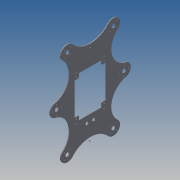
# Autodesk Inventor part: BaseAtas
Saved by Autodesk Inventor 2014 (Build 180170000, 170)
## iProperties
Created: 2014-12-20
Part Number: BaseAtas
Material: Generic
Document SubType Name: Modeling
Designer: I Was ME
Density: 1 g/cm^3
Appearance: Default
Author: I Was ME
Autodesk Inventor part; units mm, degrees
ref_plane "YZ Plane" through (0, 0, 0) normal (1, 0, 0) x (0, 1, 0)
ref_plane "XZ Plane" through (0, 0, 0) normal (0, 1, 0) x (-1, 0, 0)
ref_plane "XY Plane" through (0, 0, 0) normal (0, 0, 1) x (1, 0, 0)
sketch "Sketch1" plane through (0, 0, 0) normal (1, 0, 0) x (0, 1, 0)
  line L0 (0.007, 157.8334) -> (0.007, 7.1531) construction
  line L1 (42.757, 164.9919) -> (42.757, -0.0081) construction
  line L2 (0.007, -0.0081) -> (0.007, 164.9919) construction
  line L3 (-42.743, -0.0081) -> (-42.743, 164.9919) construction
  line L4 (-42.743, 164.9919) -> (42.757, 164.9919) construction
  line L5 (-51.5818, 156.1531) -> (-62.7081, 95.15) construction
  arc A0 (-62.7081, 95.15) -> (-51.5818, 156.1531) centre (-74.6826, 128.8502) ccw
  line L6 (-42.743, 164.9919) -> (-51.5818, 156.1531) construction
  line L7 (-42.743, 99.1738) -> (-31.743, 99.1738) construction
  line L8 (-57.145, 125.6516) -> (-39.4986, 122.433) construction
  line L9 (-42.743, 82.6501) -> (-62.743, 82.6501) construction
  arc A1 (-32.6841, 172.4128) -> (-50.4278, 155.1332) centre (-42.743, 164.9919) ccw
  circle A2 centre (-42.743, 164.9919) radius 3.5
  line L10 (42.757, -0.0081) -> (51.5959, 8.8308) construction
  arc A3 (32.6968, -7.427) -> (50.426, 9.8629) centre (42.757, -0.0081) ccw
  circle A4 centre (42.757, -0.0081) radius 3.5
  circle A5 centre (25.757, 40.7175) radius 1 construction
  line L11 (42.757, -0.0081) -> (33.9182, -8.8469) construction
  line L12 (-19.0958, -0.0081) -> (-19.0958, 82.4919) construction
  line L13 (42.757, -0.0081) -> (-42.743, -0.0081) construction
  arc A6 (33.9182, -8.8469) -> (-33.9041, -8.8469) centre (0.007, -36.7834) ccw
  line L14 (33.9182, -8.8469) -> (-33.9041, -8.8469) construction
  circle A7 centre (-25.743, 40.7175) radius 1 construction
  line L15 (42.757, 82.6501) -> (62.757, 82.6501) construction
  line L16 (62.757, 82.6501) -> (62.7799, 70.1501) construction
  line L17 (-62.743, 82.6501) -> (-62.7779, 70.1501) construction
  line L18 (-62.743, 82.6501) -> (-62.7081, 95.15) construction
  circle A8 centre (-62.743, 82.6501) radius 3.5
  arc A9 (-62.7081, 95.15) -> (-62.7779, 70.1501) centre (-62.743, 82.6501) ccw
  arc A10 (-50.4152, 9.8604) -> (-32.6827, -7.427) centre (-42.743, -0.0081) ccw
  arc A11 (-51.5818, 8.8308) -> (-62.7779, 70.1501) centre (-74.7696, 36.2788) ccw
  line L19 (-42.743, -0.0081) -> (-33.9041, -8.8469) construction
  line L20 (-42.743, -0.0081) -> (-51.5818, 8.8308) construction
  circle A12 centre (-42.743, -0.0081) radius 3.5
  line L21 (-42.743, 82.6501) -> (42.757, 82.6501) construction
  line L22 (42.757, 99.1738) -> (31.757, 99.1738) construction
  line L23 (-51.5818, 8.8308) -> (-62.7779, 70.1501) construction
  line L24 (-57.1798, 39.4904) -> (-39.4225, 42.7327) construction
  arc A13 (62.7799, 70.1501) -> (51.5959, 8.8308) centre (74.7764, 36.2824) ccw
  line L25 (62.7799, 70.1501) -> (51.5959, 8.8308) construction
  line L26 (57.1879, 39.4904) -> (39.43, 42.7293) construction
  circle A14 centre (0.007, 151.3334) radius 1
  line L27 (-25.743, 164.9919) -> (-25.743, 103.2952) construction
  arc A15 (-33.9041, 173.8308) -> (33.9182, 173.8308) centre (0.007, 201.7744) ccw
  line L28 (-33.9041, 173.8308) -> (33.9182, 173.8308) construction
  line L29 (42.757, 164.9919) -> (33.9182, 173.8308) construction
  arc A16 (50.4346, 155.1276) -> (32.6982, 172.4128) centre (42.757, 164.9919) ccw
  circle A17 centre (-25.743, 124.7175) radius 1 construction
  arc A18 (62.7799, 70.1501) -> (62.7342, 95.15) centre (62.757, 82.6501) ccw
  circle A19 centre (62.757, 82.6501) radius 3.5
  circle A20 centre (42.757, 164.9919) radius 3.5 construction
  line L30 (42.757, 164.9919) -> (51.5959, 156.1531) construction
  line L31 (62.757, 82.6501) -> (62.7342, 95.15) construction
  line L32 (51.5959, 156.1531) -> (62.7342, 95.15) construction
  line L33 (57.165, 125.6516) -> (39.5046, 122.427) construction
  arc A21 (51.5959, 156.1531) -> (62.7342, 95.15) centre (74.6746, 128.8486) ccw
  circle A22 centre (25.757, 116.7175) radius 1 construction
  circle A23 centre (-25.743, 116.7175) radius 1
  circle A24 centre (-25.743, 48.7175) radius 1 construction
  circle A25 centre (25.757, 48.7175) radius 1 construction
  line L34 (-28.993, 112.6501) -> (-28.993, 52.6501)
  line L35 (-20.993, 44.6501) -> (21.007, 44.6501)
  line L36 (29.007, 112.6501) -> (29.007, 52.6501)
  line L37 (-20.993, 120.6501) -> (21.007, 120.6501)
  line L38 (-28.993, 120.6501) -> (29.007, 120.6501) construction
  line L39 (29.007, 120.6501) -> (29.007, 44.6501) construction
  line L40 (29.007, 44.6501) -> (-28.993, 44.6501) construction
  line L41 (-28.993, 44.6501) -> (-28.993, 120.6501) construction
  line L42 (-28.993, 112.6501) -> (-22.993, 112.6501)
  line L43 (-20.993, 114.6501) -> (-20.993, 120.6501)
  line L44 (21.007, 120.6501) -> (21.007, 114.6501)
  line L45 (23.007, 112.6501) -> (29.007, 112.6501)
  line L46 (29.007, 52.6501) -> (23.007, 52.6501)
  line L47 (21.007, 50.6501) -> (21.007, 44.6501)
  line L48 (-20.993, 44.6501) -> (-20.993, 50.6501)
  line L49 (-22.993, 52.6501) -> (-28.993, 52.6501)
  arc A26 (-22.993, 112.6501) -> (-20.993, 114.6501) centre (-22.993, 114.6501) ccw
  arc A27 (21.007, 114.6501) -> (23.007, 112.6501) centre (23.007, 114.6501) ccw
  arc A28 (23.007, 52.6501) -> (21.007, 50.6501) centre (23.007, 50.6501) ccw
  arc A29 (-20.993, 50.6501) -> (-22.993, 52.6501) centre (-22.993, 50.6501) ccw
  line L50 (0.007, 120.6501) -> (0.007, 44.6501) construction
  line L51 (-28.993, 82.6501) -> (29.007, 82.6501) construction
  line L52 (62.757, 82.6501) -> (75.257, 82.6501) construction
  line L53 (42.757, -0.0081) -> (51.5959, -8.8469) construction
  line L54 (-42.743, -0.0081) -> (-51.5818, -8.8469) construction
  line L55 (-42.743, -0.0081) -> (-33.9041, 8.8308) construction
  line L56 (42.757, -0.0081) -> (33.9182, 8.8308) construction
  line L57 (42.757, 164.9919) -> (51.5959, 173.8308) construction
  line L58 (42.757, 164.9919) -> (33.9182, 156.1531) construction
  line L59 (-42.743, 164.9919) -> (-33.9041, 156.1531) construction
  line L60 (-33.9041, 156.1531) -> (-33.9041, 156.1531)
  circle A30 centre (-48.7541, 171.003) radius 0.75
  circle A31 centre (-36.7319, 171.003) radius 0.75
  circle A32 centre (-36.7319, 158.9808) radius 0.75
  circle A33 centre (-48.7541, 158.9808) radius 0.75
  line L61 (51.5959, 173.8308) -> (48.7681, 171.003) construction
  line L62 (51.5959, 156.1531) -> (48.7681, 158.9808) construction
  line L63 (33.9182, 156.1531) -> (36.7459, 158.9808) construction
  line L64 (33.9182, 173.8308) -> (36.7459, 171.003) construction
  circle A34 centre (36.7459, 171.003) radius 0.75
  circle A35 centre (36.7459, 158.9808) radius 0.75
  circle A36 centre (48.7681, 158.9808) radius 0.75
  circle A37 centre (48.7681, 171.003) radius 0.75
  line L65 (75.257, 82.6501) -> (71.258, 82.6501) construction
  line L66 (50.257, 82.6501) -> (54.256, 82.6501) construction
  line L67 (62.7799, 70.1501) -> (62.7726, 74.1491) construction
  line L68 (62.7342, 95.15) -> (62.7415, 91.151) construction
  line L69 (-75.243, 82.6501) -> (-70.8669, 82.6501) construction
  line L70 (-62.7081, 95.15) -> (-62.7193, 91.151) construction
  line L71 (-50.243, 82.6501) -> (-54.3925, 82.6501) construction
  line L72 (-62.7779, 70.1501) -> (-62.7667, 74.1491) construction
  line L73 (-62.7779, 70.1501) -> (-62.7646, 74.8991) construction
  line L74 (-50.243, 82.6501) -> (-54.242, 82.6501) construction
  line L75 (-75.243, 82.6501) -> (-71.244, 82.6501) construction
  circle A38 centre (-54.242, 82.6501) radius 0.75
  circle A39 centre (-62.7193, 91.151) radius 0.75
  circle A40 centre (-71.244, 82.6501) radius 0.75
  circle A41 centre (-62.7667, 74.1491) radius 0.75
  line L76 (51.5959, -8.8469) -> (48.7681, -6.0192)
  line L77 (51.5959, 8.8308) -> (48.7681, 6.003) construction
  line L78 (33.9182, 8.8308) -> (36.7459, 6.003) construction
  line L79 (33.9182, -8.8469) -> (36.7459, -6.0192) construction
  circle A42 centre (48.7681, -6.0192) radius 0.75
  circle A43 centre (36.7459, -6.0192) radius 0.75
  circle A44 centre (36.7459, 6.003) radius 0.75
  circle A45 centre (48.7681, 6.003) radius 0.75
  line L80 (-33.9041, -8.8469) -> (-36.7319, -6.0192)
  line L81 (-51.5818, -8.8469) -> (-48.7541, -6.0192) construction
  line L82 (-51.5818, 8.8308) -> (-48.7541, 6.003) construction
  line L83 (-33.9041, 8.8308) -> (-33.9041, 8.8308) construction
  line L84 (-33.9041, 8.8308) -> (-36.7319, 6.003) construction
  circle A46 centre (-36.7319, 6.003) radius 0.75
  circle A47 centre (-48.7541, 6.003) radius 0.75
  circle A48 centre (-48.7541, -6.0192) radius 0.75
  circle A49 centre (-36.7319, -6.0192) radius 0.75
  circle A50 centre (42.757, 164.9919) radius 3.5
  circle A51 centre (54.256, 82.6501) radius 0.75
  circle A52 centre (62.7726, 74.1491) radius 0.75
  circle A53 centre (71.258, 82.6501) radius 0.75
  circle A54 centre (62.7415, 91.151) radius 0.75
  circle A55 centre (-6.243, 32.1501) radius 2.75
  circle A56 centre (6.257, 32.1501) radius 2.75
  circle A57 centre (25.757, 124.7175) radius 1
  circle A58 centre (25.757, 116.7175) radius 1
  circle A59 centre (-25.743, 124.7175) radius 1
  circle A60 centre (25.757, 48.7175) radius 1
  circle A61 centre (25.757, 40.7175) radius 1
  circle A62 centre (-25.743, 40.7175) radius 1
  circle A63 centre (-25.743, 48.7175) radius 1
  point P0 (0, 0)
  point P1 (0, 0)
  point P2 (0.007, 82.6501)
  point P3 (6.257, 32.1501)
  dimension "d0" = 165
  dimension "d1" = 85.5
  dimension "d2" = 82.5
  dimension "d3" = 20
  dimension "d4" = 20
  dimension "d5" = 25
  dimension "d6" = 25
  dimension "d7" = 25
  dimension "d8" = 25
  dimension "d9" = 25
  dimension "d10" = 25
  dimension "d11" = 7
  dimension "d12" = 7
  dimension "d13" = 7
  dimension "d14" = 7
  dimension "d15" = 7
  dimension "d16" = 7
  dimension "d17" = 45
  dimension "d18" = 45
  dimension "d19" = 45
  dimension "d20" = 45
  dimension "d21" = 45
  dimension "d22" = 45
  dimension "d23" = 45
  dimension "d24" = 90
  dimension "d27" = 11
  dimension "d28" = 11
  dimension "d29" = 150.6803
  dimension "d30" = 61.6967
  dimension "d43" = 2
  dimension "d44" = 6.5
  dimension "d46" = 2
  dimension "d49" = 17
  dimension "d51" = 2
  dimension "d52" = 2
  dimension "d55" = 17
  dimension "d56" = 17
  dimension "d57" = 2
  dimension "d58" = 2
  dimension "d59" = 8
  dimension "d61" = 2
  dimension "d62" = 8
  dimension "d63" = 2
  dimension "d64" = 8
  dimension "d67" = 42
  dimension "d70" = 58
  dimension "d71" = 76
  dimension "d72" = 2
  dimension "d76" = 12.5
  dimension "d78" = 36.5
  dimension "d79" = 90
  dimension "d80" = 90
  dimension "d81" = 90
  dimension "d82" = 90
  dimension "d88" = 1.5
  dimension "d89" = 1.5
  dimension "d90" = 1.5
  dimension "d91" = 1.5
  dimension "d92" = 1.5
  dimension "d93" = 1.5
  dimension "d94" = 1.5
  dimension "d95" = 1.5
  dimension "d96" = 3.999
  dimension "d97" = 3.999
  constraints: 170 end point, 64 centre point, 60 point on circle, 37 point on line, 36 coincident, 20 perpendicular, 16 midpoint, 14 parallel, 8 collinear, 8 tangent, 3 equal radius, 2 horizontal, 1 equal length
  measures "d0" distance of L3.start L3.end
  measures "d1" distance of L1.end L3.start
  measures "d2" distance of L12.start L12.end
  measures "d3" distance of L21.start L9.end
  measures "d4" distance of L21.end L15.end
  measures "d5" diameter of A9
  measures "d6" diameter of A18
  measures "d7" diameter of A16
  measures "d8" diameter of A1
  measures "d9" diameter of A3
  measures "d10" diameter of A10
  measures "d11" diameter of A12
  measures "d12" diameter of A4
  measures "d13" diameter of A19
  measures "d14" diameter of A8
  measures "d15" diameter of A20
  measures "d16" diameter of A2
  measures "d17" angle of L4 L29
  measures "d18" angle of L1 L30
  measures "d19" angle of L3 L6
  measures "d20" angle of L3 L20
  measures "d21" angle of L13 L19
  measures "d22" angle of L1 L10
  measures "d23" angle of L13 L11
  measures "d24" angle of L23 L24
  measures "d27" distance of L7.start L7.end
  measures "d28" distance of L22.start L22.end
  measures "d29" distance of L0.start L0.end
  measures "d30" distance of L27.start L27.end
  measures "d43" diameter of A14
  measures "d44" distance of A14.centre L0.start
  measures "d46" diameter of A17
  measures "d49" distance from line of L3 A17.centre
  measures "d51" diameter of A5
  measures "d52" diameter of A7
  measures "d55" distance from line of L3 A7.centre
  measures "d56" distance from line of L1 A5.centre
  measures "d57" diameter of A23
  measures "d58" diameter of A22
  measures "d59" distance of A23.centre A17.centre
  measures "d61" diameter of A24
  measures "d62" distance of A7.centre A24.centre
  measures "d63" diameter of A25
  measures "d64" distance of A5.centre A25.centre
  measures "d67" distance of L35.start L35.end
  measures "d70" distance of L38.start L38.end
  measures "d71" distance of L38.end L39.end
  measures "d72" radius of A26
  measures "d76" distance from line of L35 point (6.257, 32.15)
  measures "d78" distance from line of L1 point (6.257, 32.15)
  measures "d79" angle of L11 L53
  measures "d80" angle of L19 L54
  measures "d81" angle of L30 L57
  measures "d82" angle of L58 L29
  measures "d88" diameter of A30
  measures "d89" diameter of A31
  measures "d90" diameter of A32
  measures "d91" diameter of A33
  measures "d92" diameter of A34
  measures "d93" diameter of A37
  measures "d94" diameter of A36
  measures "d95" diameter of A35
  measures "d96" distance of L52.end L65.end
  measures "d97" distance of L66.start L66.end
sketch "Sketch2" plane through (0, 0, 0) normal (1, 0, 0) x (0, 1, 0)
  point P0 (0, 0)
sketch "Sketch3" plane through (0, 0, 0) normal (1, 0, 0) x (0, 1, 0)
  point P0 (0, 0)
sketch "Sketch4" plane through (0, 0, 0) normal (1, 0, 0) x (0, 1, 0)
  point P0 (0, 0)
sketch "Sketch5" plane through (0, 0, 0) normal (1, 0, 0) x (0, 1, 0)
  point P0 (0, 0)
extrude "Extrusion1" add sketch "Sketch1" along normal blind 1.5 contours A0 A1 A15 A16 A21 A18 A13 A3 A6 A10 A11 A9
body "Solid1"
